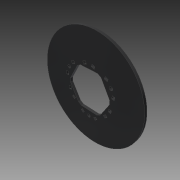
# Autodesk Inventor part: spool_b
Saved by Autodesk Inventor 2014 (Build 180170000, 170)
## iProperties
Created: 2014-04-05
Part Number: spool_b
Material: Plywood, Finish
Document SubType Name: Modeling
Designer: buben
Density: 0.552 g/cm^3
Appearance: Anodized - Dark Gray
Author: buben
Autodesk Inventor part; units mm, degrees
ref_plane "YZ Plane" through (0, 0, 0) normal (1, 0, 0) x (0, 1, 0)
ref_plane "XZ Plane" through (0, 0, 0) normal (0, 1, 0) x (-1, 0, 0)
ref_plane "XY Plane" through (0, 0, 0) normal (0, 0, 1) x (1, 0, 0)
sketch "Sketch1" plane through (0, 0, 0) normal (0, 1, 0) x (-1, 0, 0)
  circle A0 centre (0, 0) radius 75 construction
  line L0 (67.7446, 23.8956) -> (61.3434, 25.0243) construction
  line L1 (61.3434, 25.0243) -> (51.7927, -29.1401) construction
  line L2 (51.7927, -29.1401) -> (58.194, -30.2688) construction
  line L3 (58.194, -30.2688) -> (67.7446, 23.8956) construction
  line L4 (55.3106, -35.2631) -> (51.1324, -30.2838) construction
  line L5 (51.1324, -30.2838) -> (9, -65.6371) construction
  line L6 (9, -65.6371) -> (13.1781, -70.6164) construction
  line L7 (13.1781, -70.6164) -> (55.3106, -35.2631) construction
  line L8 (-13.1781, -70.6164) -> (-9, -65.6371) construction
  line L9 (-9, -65.6371) -> (-51.1324, -30.2838) construction
  line L10 (-51.1324, -30.2838) -> (-55.3106, -35.2631) construction
  line L11 (-55.3106, -35.2631) -> (-13.1781, -70.6164) construction
  line L12 (-58.194, -30.2688) -> (-51.7927, -29.1401) construction
  line L13 (-51.7927, -29.1401) -> (-61.3434, 25.0243) construction
  line L14 (-61.3434, 25.0243) -> (-67.7446, 23.8956) construction
  line L15 (-67.7446, 23.8956) -> (-58.194, -30.2688) construction
  line L16 (52.3434, 40.6128) -> (54.5665, 46.7208) construction
  line L17 (54.5665, 46.7208) -> (2.8834, 65.5319) construction
  line L18 (2.8834, 65.5319) -> (0.6603, 59.4239) construction
  line L19 (0.6603, 59.4239) -> (52.3434, 40.6128) construction
  line L20 (-0.6603, 59.4239) -> (-2.8834, 65.5319) construction
  line L21 (-2.8834, 65.5319) -> (-54.5665, 46.7208) construction
  line L22 (-54.5665, 46.7208) -> (-52.3434, 40.6128) construction
  line L23 (-52.3434, 40.6128) -> (-0.6603, 59.4239) construction
  line L24 (9, -65.6371) -> (61.3434, 25.0243) construction
  line L25 (52.3434, 40.6128) -> (-52.3434, 40.6128) construction
  line L26 (-61.3434, 25.0243) -> (-9, -65.6371) construction
  arc A1 (67.7446, 23.8956) -> (54.5665, 46.7208) centre (45.8993, 26.5) ccw construction
  arc A2 (-13.1781, -70.6164) -> (13.1781, -70.6164) centre (0, -53) ccw construction
  arc A3 (-54.5665, 46.7208) -> (-67.7446, 23.8956) centre (-45.8993, 26.5) ccw construction
  circle A4 centre (56.2917, 32.5) radius 4.25
  circle A5 centre (0, 0) radius 132.5
  line L27 (-22.8675, 50) -> (22.8675, 50)
  line L28 (31.8675, 44.8038) -> (54.735, 5.1962)
  line L29 (54.735, -5.1962) -> (31.8675, -44.8038)
  line L30 (22.8675, -50) -> (-22.8675, -50)
  line L31 (-31.8675, -44.8038) -> (-54.735, -5.1962)
  line L32 (-54.735, 5.1962) -> (-31.8675, 44.8038)
  line L33 (54.735, -5.1962) -> (54.735, 5.1962)
  line L34 (31.8675, 44.8038) -> (22.8675, 50)
  line L35 (-22.8675, 50) -> (-31.8675, 44.8038)
  line L36 (-54.735, 5.1962) -> (-54.735, -5.1962)
  line L37 (-31.8675, -44.8038) -> (-22.8675, -50)
  line L38 (22.8675, -50) -> (31.8675, -44.8038)
  line L39 (45.8993, 26.5) -> (0, 0) construction
  line L40 (0, 0) -> (0, -53) construction
  line L41 (0, 0) -> (-45.8993, 26.5) construction
  circle A6 centre (0, -65) radius 4.25
  circle A7 centre (-56.2917, 32.5) radius 4.25
  line L42 (-60.3015, 19.1155) -> (-58.9123, 11.237)
  line L43 (-58.9123, 11.237) -> (-65.3136, 10.1083)
  line L44 (-65.3136, 10.1083) -> (-66.7028, 17.9868)
  line L45 (-66.7028, 17.9868) -> (-60.3015, 19.1155)
  line L46 (-19.7246, -56.6381) -> (-13.5963, -61.7804)
  line L47 (-13.5963, -61.7804) -> (-17.7744, -66.7597)
  line L48 (-17.7744, -66.7597) -> (-23.9027, -61.6174)
  line L49 (-23.9027, -61.6174) -> (-19.7246, -56.6381)
  line L50 (50.7143, -39.1198) -> (44.5859, -44.2621)
  line L51 (44.5859, -44.2621) -> (40.4078, -39.2828)
  line L52 (40.4078, -39.2828) -> (46.5362, -34.1405)
  line L53 (46.5362, -34.1405) -> (50.7143, -39.1198)
  line L54 (-46.5362, -34.1405) -> (-40.4078, -39.2828)
  line L55 (-40.4078, -39.2828) -> (-44.5859, -44.2621)
  line L56 (-44.5859, -44.2621) -> (-50.7143, -39.1198)
  line L57 (-50.7143, -39.1198) -> (-46.5362, -34.1405)
  line L58 (-54.2238, -15.3528) -> (-52.8346, -23.2313)
  line L59 (-52.8346, -23.2313) -> (-59.2359, -24.36)
  line L60 (-59.2359, -24.36) -> (-60.6251, -16.4815)
  line L61 (-60.6251, -16.4815) -> (-54.2238, -15.3528)
  line L62 (-16.0391, 60.7436) -> (-8.5216, 63.4798)
  line L63 (-8.5216, 63.4798) -> (-6.2985, 57.3718)
  line L64 (-6.2985, 57.3718) -> (-13.816, 54.6356)
  line L65 (-13.816, 54.6356) -> (-16.0391, 60.7436)
  line L66 (-48.9284, 48.7729) -> (-41.4108, 51.5091)
  line L67 (-41.4108, 51.5091) -> (-39.1877, 45.4011)
  line L68 (-39.1877, 45.4011) -> (-46.7052, 42.6649)
  line L69 (-46.7052, 42.6649) -> (-48.9284, 48.7729)
  line L70 (8.5216, 63.4798) -> (16.0391, 60.7436)
  line L71 (16.0391, 60.7436) -> (13.816, 54.6356)
  line L72 (13.816, 54.6356) -> (6.2985, 57.3718)
  line L73 (6.2985, 57.3718) -> (8.5216, 63.4798)
  line L74 (41.4108, 51.5091) -> (48.9284, 48.7729)
  line L75 (48.9284, 48.7729) -> (46.7052, 42.6649)
  line L76 (46.7052, 42.6649) -> (39.1877, 45.4011)
  line L77 (39.1877, 45.4011) -> (41.4108, 51.5091)
  line L78 (66.7028, 17.9868) -> (65.3136, 10.1083)
  line L79 (65.3136, 10.1083) -> (58.9123, 11.237)
  line L80 (58.9123, 11.237) -> (60.3015, 19.1155)
  line L81 (60.3015, 19.1155) -> (66.7028, 17.9868)
  line L82 (60.6251, -16.4815) -> (59.2359, -24.36)
  line L83 (59.2359, -24.36) -> (52.8346, -23.2313)
  line L84 (52.8346, -23.2313) -> (54.2238, -15.3528)
  line L85 (54.2238, -15.3528) -> (60.6251, -16.4815)
  line L86 (23.9027, -61.6174) -> (17.7744, -66.7597)
  line L87 (17.7744, -66.7597) -> (13.5963, -61.7804)
  line L88 (13.5963, -61.7804) -> (19.7246, -56.6381)
  line L89 (19.7246, -56.6381) -> (23.9027, -61.6174)
  circle A8 centre (56.2917, 32.5) radius 14 construction
  circle A9 centre (-56.2917, 32.5) radius 14 construction
  circle A10 centre (0, -65) radius 14 construction
  point P0 (-28.8675, 50)
  point P1 (28.8675, 50)
  point P2 (57.735, 0)
  point P3 (28.8675, -50)
  point P4 (-28.8675, -50)
  point P5 (-57.735, 0)
  dimension "d0" = 150
  dimension "d8" = 6.5
  dimension "d9" = 18
  dimension "d10" = 18
  dimension "d11" = 18
  dimension "d13" = 60
  dimension "d14" = 20
  dimension "d15" = 20
  dimension "d16" = 20
  dimension "d17" = 20
  dimension "d18" = 20
  dimension "d19" = 20
  dimension "d21" = 60
  dimension "d23" = 22
  dimension "d24" = 8.5
  dimension "d25" = 265
  dimension "d26" = 55
  dimension "d27" = 6
  dimension "d28" = 6
  dimension "d29" = 6
  dimension "d30" = 6
  dimension "d31" = 6
  dimension "d32" = 6
  dimension "d33" = 6
  dimension "d34" = 6
  dimension "d35" = 6
  dimension "d36" = 6
  dimension "d37" = 6
  dimension "d38" = 6
  dimension "d39" = 65
  dimension "d40" = 50
  dimension "d41" = 65
  dimension "d42" = 65
  dimension "d43" = 6.5
  dimension "d44" = 8
  dimension "d45" = 6
  dimension "d46" = 6
  dimension "d47" = 6
  dimension "d48" = 6
  dimension "d49" = 6
  dimension "d50" = 6
  dimension "d51" = 6
  dimension "d52" = 6
  dimension "d53" = 6
  dimension "d54" = 6
  dimension "d55" = 6
  dimension "d56" = 6
  dimension "d62" = 28
  constraints: 180 end point, 36 parallel, 34 equal length, 18 perpendicular, 15 point on line, 12 collinear, 11 centre point, 6 coincident, 6 equal radius, 6 point on circle, 3 tangent, 2 horizontal, 1 horizontal alignment, 13 other
  measures "d0" diameter of A0
  measures "d8" distance of L16.start L16.end
  measures "d9" distance of L16.start L0.end
  measures "d10" distance of L13.end L22.end
  measures "d11" distance of L8.end L5.end
  measures "d13" angle of L25 L26
  measures "d14" angle of L24 L5
  measures "d15" angle of L24 L1
  measures "d16" angle of L25 L23
  measures "d17" angle of L26 L13
  measures "d18" angle of L26 L9
  measures "d19" angle of L25 L19
  measures "d21" angle of L25 L24
  measures "d23" radius of A1
  measures "d24" diameter of A4
  measures "d25" diameter of A5
  measures "d26" distance of L16.end L17.end
  measures "d27" distance of L29.start point (57.735, 0)
  measures "d28" distance of L28.end point (57.735, 0)
  measures "d29" distance of L28.start point (28.868, 50)
  measures "d30" distance of L27.end point (28.868, 50)
  measures "d31" distance of L27.start point (-28.868, 50)
  measures "d32" distance of L32.end point (-28.868, 50)
  measures "d33" distance of L32.start point (-57.735, 0)
  measures "d34" distance of L31.end point (-57.735, 0)
  measures "d35" distance of L31.start point (-28.868, -50)
  measures "d36" distance of L30.end point (-28.868, -50)
  measures "d37" distance of L30.start point (28.868, -50)
  measures "d38" distance of L29.end point (28.868, -50)
  measures "d39" distance of point (0, 0) A4.centre
  measures "d40" distance from line of L27 point (0, 0)
  measures "d41" distance of A7.centre point (0, 0)
  measures "d42" distance of point (0, 0) A6.centre
  measures "d43" distance of L44.end L42.start
  measures "d44" distance of L43.end L44.end
  measures "d45" distance between parallel lines of L0 L81
  measures "d46" distance between parallel lines of L2 L83
  measures "d47" distance between parallel lines of L4 L53
  measures "d48" distance between parallel lines of L6 L87
  measures "d49" distance between parallel lines of L16 L75
  measures "d50" distance between parallel lines of L73 L18
  measures "d51" distance between parallel lines of L20 L63
  measures "d52" distance between parallel lines of L22 L69
  measures "d53" distance between parallel lines of L14 L45
  measures "d54" distance between parallel lines of L12 L59
  measures "d55" distance between parallel lines of L10 L57
  measures "d56" distance between parallel lines of L8 L47
  measures "d62" diameter of A8
extrude "Extrusion1" add sketch "Sketch1" along normal blind 6.5
equation "\"d15\" = d14"
equation "\"d16\" = d15"
equation "\"d17\" = d15"
equation "\"d18\" = d15"
equation "\"d19\" = d15"
equation "\"d28\" = d27"
equation "\"d29\" = d27"
equation "\"d30\" = d29"
equation "\"d31\" = d27"
equation "\"d32\" = d31"
equation "\"d33\" = d27"
equation "\"d34\" = d33"
equation "\"d35\" = d27"
equation "\"d36\" = d35"
equation "\"d37\" = d27"
equation "\"d38\" = d37"
body "Solid1"
